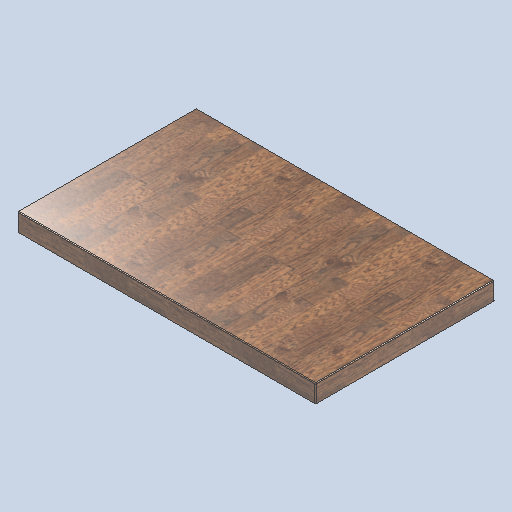
# Autodesk Inventor part: Top Panel
Saved by Autodesk Inventor 2022 (Build 260153000, 153)
## iProperties
RuleStatus: InUse
Created: 2021-10-04
Part Number: Top Panel
Material: Generic
Document SubType Name: Modeling
Designer: Admin
Density: 1 g/cm^3
Appearance: White Ash - Java
Author: Admin
Autodesk Inventor part; units mm, degrees
ref_plane "YZ Plane" through (0, 0, 0) normal (1, 0, 0) x (0, 1, 0)
ref_plane "XZ Plane" through (0, 0, 0) normal (0, 1, 0) x (-1, 0, 0)
ref_plane "XY Plane" through (0, 0, 0) normal (0, 0, 1) x (1, 0, 0)
derived "Dresser SKELETON.ipt"
sketch "Top Sketch" plane through (0, 1219.2, 0) normal (0, 1, 0) x (-1, 0, 0)
  line L0 (635, 381) -> (635, -381)
  line L1 (635, -381) -> (-635, -381)
  line L2 (-635, 381) -> (635, 381)
  line L3 (-635, -381) -> (-635, 381)
  point P0 (0, 0)
extrude "Extrusion1" add sketch "Top Sketch" against normal blind 76.2
fillet "Fillet1" radius 3.175 8 edges at (-635, 1181.1, 381) (0, 1219.2, 381) (635, 1181.1, 381) (635, 1219.2, 0) (-635, 1219.2, 0) (635, 1181.1, -381) (0, 1219.2, -381) (-635, 1181.1, -381)
sketch "Sketch3" plane through (0, 1219.2, 457.2) normal (1, 0, 0) x (0, 0, -1)
  line L0 (76.2, -76.2) -> (95.25, -57.15)
  line L1 (95.25, -57.15) -> (86.1102, -48.0102)
  line L2 (86.1102, -41.6602) -> (95.25, -32.5204)
  arc A0 (108.7204, 0) -> (95.25, -32.5204) centre (108.7204, -19.05) ccw
  line L3 (76.2, 0) -> (76.2, -76.2)
  line L4 (76.2, -76.2) -> (76.2, 0)
  line L5 (76.2, 0) -> (108.7204, 0)
  line L6 (86.1102, -48.0102) -> (86.1102, -41.6602)
  dimension "d6" = 6.35
  dimension "d7" = 19.05
  dimension "d12" = 45
  dimension "d13" = 76.2
  dimension "d14" = 19.05
  constraints: 12 end point, 3 perpendicular, 2 point on circle, 1 centre point, 1 coincident, 1 line through centre, 1 tangent, 1 vertical, 1 vertical alignment, 3 other
  measures "d6" distance of L1.end L2.start
  measures "d7" radius of A0
  measures "d12" angle to the sketch x axis of L0
  measures "d13" distance of L4.end L0.start
  measures "d14" horizontal distance of L0.end L0.start
feature "Elegant Sweep" [suppressed]
fillet "Elegant Fillet" [suppressed]
equation "\"d1\" = topThickness"
equation "\"d7\" = d14"
equation "\"d13\" = topThickness"
equation "\"d14\" = 0.25 * topThickness"
equation "\"topThickness\" = 76.2"
body "Solid1"
